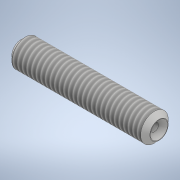
# Autodesk Inventor part: throat
Saved by Autodesk Inventor 2020.2 (Build 242310000, 310)
## iProperties
Created: 2017-11-12
Part Number: throat
Material: Ogólny
Document SubType Name: Modeling
Designer: Haras
Density: 1 g/cm^3
Appearance: Domyślna
Author: Haras
Autodesk Inventor part; units mm, degrees
ref_plane "YZ Plane" through (0, 0, 0) normal (1, 0, 0) x (0, 1, 0)
ref_plane "XZ Plane" through (0, 0, 0) normal (0, 1, 0) x (-1, 0, 0)
ref_plane "XY Plane" through (0, 0, 0) normal (0, 0, 1) x (1, 0, 0)
sketch "Szkic1" plane through (0, 0, 0) normal (1, 0, 0) x (0, 1, 0)
  circle A0 centre (0, 0) radius 3
  dimension "d0" = 6
  constraints: 1 centre point, 1 coincident
  measures "d0" diameter of A0
extrude "Wyciągnięcie proste1" add sketch "Szkic1" along normal blind 30
sketch "Szkic2" plane through (30, 0, 0) normal (1, 0, 0) x (0, 0, -1)
  point P0 (0, 0)
  point P1 (0, 0)
  constraints: 1 coincident
hole "Otwór1" at (30, 0, 0) direction (-1, 0, 0) diameter 1.75 end through all
thread "Gwint1" size "M6x1" class "6g" standard "ANSI Metric M Profile" full length
chamfer "Faza1" distance 1 angle 45 2 edges at (30, -3, 0) (0, -3, 0)
chamfer "Faza2" distance 1 angle 45 1 edges at (30, 0, 0.875)
